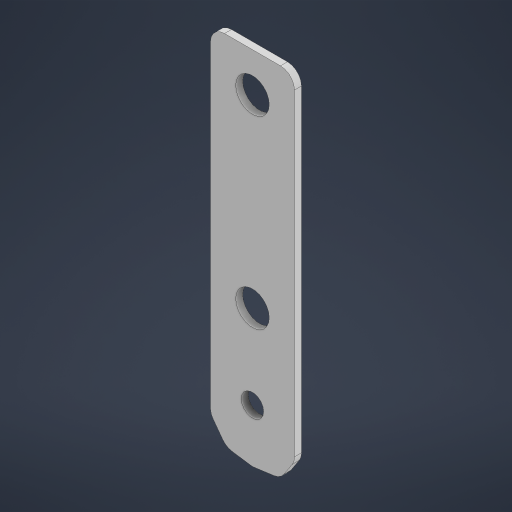
# Autodesk Inventor part: PTOPoly
Saved by Autodesk Inventor 2023.4 (Build 274418000, 418)
## iProperties
Created: 2024-03-12
Part Number: PTOPoly
Material: Generic
Document SubType Name: Modeling
Designer: Meer
Density: 1 g/cm^3
Appearance: Default
Author: Meer
Autodesk Inventor part; units mm, degrees
ref_plane "YZ Plane" through (0, 0, 0) normal (1, 0, 0) x (0, 1, 0)
ref_plane "XZ Plane" through (0, 0, 0) normal (0, 1, 0) x (-1, 0, 0)
ref_plane "XY Plane" through (0, 0, 0) normal (0, 0, 1) x (1, 0, 0)
sketch "Sketch1" plane through (0, 0, 0) normal (0, 0, 1) x (1, 0, 0)
  line L0 (0, 0) -> (12.7, 0)
  line L1 (9.525, 0) -> (9.525, 76.2)
  line L2 (9.525, 76.2) -> (-9.525, 76.2)
  line L3 (-9.525, 76.2) -> (-9.525, 0)
  line L4 (-9.525, 0) -> (0, -5.7165)
  line L5 (0, -5.7165) -> (9.525, 0)
  line L6 (-9.525, 0) -> (-5.9562, -4.8471)
  line L7 (-5.9562, -4.8471) -> (0, -5.7165)
  line L8 (0, -5.7165) -> (6.35, -4.8471)
  line L9 (6.35, -4.8471) -> (9.525, 0)
  line L10 (-9.525, 0) -> (0, 0)
  line L11 (0, 0) -> (0, 6.35)
  line L12 (0, 6.35) -> (0, 25.4)
  circle A0 centre (0, 25.4) radius 3.81
  circle A1 centre (0, 6.35) radius 2.54
  line L13 (0, 21.59) -> (0, 8.89)
  line L14 (0, 29.21) -> (0, 67.31)
  circle A2 centre (0, 67.31) radius 3.81
  dimension "d29" = 5.08
  dimension "d7" = 76.2
  dimension "d22" = 6.35
  dimension "d23" = 19.05
  dimension "d28" = 7.62
  dimension "d30" = 38.1
  dimension "d31" = 7.62
  constraints: 30 end point, 6 point on line, 3 coincident, 2 centre point, 2 horizontal, 2 point on circle, 1 parallel, 1 perpendicular, 1 vertical alignment, 2 other
  measures "d7" distance of L1.end L1.start
  measures "d22" distance of L0.start L11.end
  measures "d23" distance of L11.end L12.end
  measures "d28" diameter of A0
  measures "d30" distance of L14.start L14.end
  measures "d31" diameter of A2
extrude "Extrusion5" add sketch "Sketch1" along normal blind 1.5875
fillet "Fillet4" radius 3.175 7 edges at (6.35, -4.8471, 0.7937) (9.525, 0, 0.7937) (0, -5.7165, 0.7937) (-5.9562, -4.8471, 0.7937) (-9.525, 0, 0.7937) (9.525, 76.2, 0.7937) (-9.525, 76.2, 0.7937)
body "Solid5"
